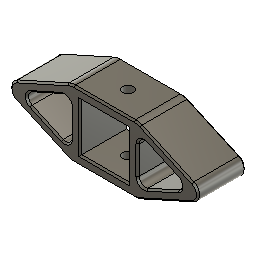
Extrusion_Wrench_1515 (Autodesk Fusion 360 design; units mm, degrees)
Autodesk Fusion 360 part; units mm, degrees
sketch "Sketch1" plane through (0, 0, 0) normal (0, 0, 1) x (1, 0, 0)
  line L0 (10.5, 10.5) -> (-10.5, 10.5)
  line L1 (-10.5, 10.5) -> (-10.5, -10.5)
  line L2 (-10.5, -10.5) -> (10.5, -10.5)
  line L3 (10.5, -10.5) -> (10.5, 10.5)
  line L4 (10.5, 10.5) -> (-10.5, -10.5) construction
  line L5 (-10.5, 10.5) -> (10.5, -10.5) construction
  line L6 (7.5, 7.5) -> (-7.5, 7.5)
  line L7 (-7.5, 7.5) -> (-7.5, -7.5)
  line L8 (-7.5, -7.5) -> (7.5, -7.5)
  line L9 (7.5, -7.5) -> (7.5, 7.5)
  line L10 (7.5, 7.5) -> (-7.5, -7.5) construction
  line L11 (-7.5, 7.5) -> (7.5, -7.5) construction
  line L12 (10.5, 10.5) -> (27.7245, 2.7349)
  line L13 (27.7245, -2.7349) -> (10.5, -10.5)
  line L14 (-10.5, 10.5) -> (-27.7245, 2.7349)
  line L15 (-27.7245, -2.7349) -> (-10.5, -10.5)
  arc A0 (27.7245, -2.7349) -> (27.7245, 2.7349) centre (26.4916, 0) ccw
  arc A1 (-27.7245, 2.7349) -> (-27.7245, -2.7349) centre (-26.4916, 0) ccw
  line L16 (26.4916, 0) -> (0, 0) construction
  line L17 (0, 0) -> (-26.4916, 0) construction
  line L18 (7.5, 7.5) -> (10.5, 7.5) construction
  line L19 (7.5, -7.5) -> (10.5, -7.5) construction
  line L20 (-7.5, -7.5) -> (-10.5, -7.5) construction
  line L21 (-7.5, 7.5) -> (-10.5, 7.5) construction
  line L22 (10.5, 7.5) -> (27.1365, 0)
  line L23 (10.5, -7.5) -> (27.1365, 0)
  line L24 (-10.5, 7.5) -> (-27.1365, 0)
  line L25 (-10.5, -7.5) -> (-27.1365, 0)
  line L26 (-24.3008, 1.2784) -> (-24.3008, -1.2784)
  line L27 (24.3008, -1.2784) -> (24.3008, 1.2784)
  dimension "d1" = 15
  dimension "d2" = 3
  dimension "d3" = 3
  dimension "d4" = 3
  constraint horizontal L0
  constraint perpendicular L0 L1
  constraint parallel L0 L2
  constraint parallel L1 L3
  constraint coincident L4 L16.end
  constraint coincident L5 L16.end
  constraint coincident L16.end L17.start
  constraint horizontal L6
  constraint perpendicular L6 L7
  constraint parallel L6 L8
  constraint parallel L7 L9
  constraint coincident L4 L6.start
  constraint coincident L10 L16.end
  constraint coincident L11 L16.end
  constraint equal L6 L9
  constraint tangent L13 A0
  constraint tangent L12 A0
  constraint tangent L15 A1
  constraint tangent L14 A1
  constraint equal L12 L14
  constraint coincident A0.centre L16.start
  constraint coincident A1.centre L17.end
  constraint horizontal L17
  constraint horizontal L16
  constraint coincident L3 L18.end
  constraint perpendicular L3 L18
  constraint coincident L3 L19.end
  constraint perpendicular L3 L19
  constraint coincident L1 L20.end
  constraint perpendicular L1 L20
  constraint perpendicular L1 L21
  constraint coincident L1 L21.end
  constraint coincident L16 L22.end
  constraint parallel L12 L22
  constraint coincident L17 L24.end
  constraint equal L22 L24
  constraint coincident L24 L26.start
  constraint coincident L25 L26.end
  constraint perpendicular L17 L26
  constraint coincident L23 L27.start
  constraint coincident L22 L27.end
  constraint parallel L26 L27
  constraint equal L26 L27
  measures "d1" distance of L6.start L6.end
  measures "d2" distance of L0 L6
  measures "d3" radius of A0
  measures "d4" radius of A1
extrude "Extrude1" add sketch "Sketch1" along normal blind 15 contours L0 L1 L2 L3 | L3 L12 L13 A0 L22 L23 | L1 L14 L15 A1 L24 L25 | L22 L23 L27 | L24 L25 L26
fillet "Fillet1" radius 5 4 edges at (-10.5, -10.5, 7.5) (10.5, -10.5, 7.5) (10.5, 10.5, 7.5) (-10.5, 10.5, 7.5)
fillet "Fillet2" radius 2 8 edges at (-10.5, 7.5, 7.5) (-10.5, -7.5, 7.5) (-24.3008, -1.2784, 7.5) (-24.3008, 1.2784, 7.5) (10.5, 7.5, 7.5) (10.5, -7.5, 7.5) (24.3008, -1.2784, 7.5) (24.3008, 1.2784, 7.5)
sketch "Sketch2" plane through (0, 10.5, 0) normal (0, 1, 0) x (-1, 0, 0)
  line L0 (9.4251, 0) -> (9.4251, 15)
  line L1 (9.4251, 15) -> (-9.4251, 15)
  line L2 (-9.4251, 15) -> (-9.4251, 0)
  line L3 (-9.4251, 0) -> (9.4251, 0)
  circle A0 centre (0, 7.5) radius 1.65
  dimension "d13" = 3.3
  measures "d13" diameter of A0
extrude "Extrude2" cut sketch "Sketch2" against normal blind 35 contours A0
chamfer "Chamfer1" distance 0.5 angle 45 2 faces at (2.5, -9.5, 0) (2.5, -9.5, 15)
named bodies: "Extrusion_Wrench_1515"
